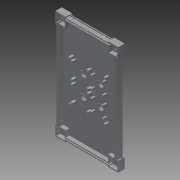
# Autodesk Inventor part: SimpleLensPlane
Saved by Autodesk Inventor 2015 (Build 190159000, 159)
## iProperties
Created: 2015-03-20
Part Number: SimpleLensPlane
Material: NylonD2W
Document SubType Name: Modeling
Designer: Akovo_000
Density: 0.93 g/cm^3
Appearance: Nylon 6
Mass: 59.4864 g
Surface Area: 763.227 cm^2
Volume: 63.9639 cm^3
Author: Akovo_000
Autodesk Inventor part; units mm, degrees
ref_plane "YZ Plane" through (0, 0, 0) normal (1, 0, 0) x (0, 1, 0)
ref_plane "XZ Plane" through (0, 0, 0) normal (0, 1, 0) x (-1, 0, 0)
ref_plane "XY Plane" through (0, 0, 0) normal (0, 0, 1) x (1, 0, 0)
ref_plane "Main Work Pane" through (0, 2.75, 7) normal (0, 1, 0) x (-1, 0, 0)
sketch "Panel" plane through (0, 2.75, 7) normal (0, 1, 0) x (-1, 0, 0)
  circle A0 centre (9.4297, 27.3549) radius 5.8
  circle A1 centre (9.4297, -11.6451) radius 5.8
  circle A2 centre (43.2297, -11.6451) radius 5.8
  circle A3 centre (43.2297, 27.3549) radius 5.8
  line L0 (43.2297, -11.6451) -> (43.2297, -11.6451)
  line L1 (61.2297, 45.3549) -> (25.2297, 45.3549)
  line L2 (25.2297, 45.3549) -> (25.2297, 9.3549)
  line L3 (25.2297, 9.3549) -> (61.2297, 9.3549)
  line L4 (61.2297, 9.3549) -> (61.2297, 45.3549)
  line L5 (61.2297, 45.3549) -> (25.2297, 9.3549) construction
  line L6 (25.2297, 45.3549) -> (61.2297, 9.3549) construction
  line L7 (61.2297, 6.3549) -> (25.2297, 6.3549)
  line L8 (25.2297, 6.3549) -> (25.2297, -29.6451)
  line L9 (25.2297, -29.6451) -> (61.2297, -29.6451)
  line L10 (61.2297, -29.6451) -> (61.2297, 6.3549)
  line L11 (61.2297, 6.3549) -> (25.2297, -29.6451) construction
  line L12 (25.2297, 6.3549) -> (61.2297, -29.6451) construction
  line L13 (22.2297, 40.1549) -> (-3.3703, 40.1549)
  line L14 (-3.3703, 40.1549) -> (-3.3703, 14.5549)
  line L15 (-3.3703, 14.5549) -> (22.2297, 14.5549)
  line L16 (22.2297, 14.5549) -> (22.2297, 40.1549)
  line L17 (22.2297, 40.1549) -> (-3.3703, 14.5549) construction
  line L18 (-3.3703, 40.1549) -> (22.2297, 14.5549) construction
  line L19 (22.2297, 1.1549) -> (-3.3703, 1.1549)
  line L20 (-3.3703, 1.1549) -> (-3.3703, -24.4451)
  line L21 (-3.3703, -24.4451) -> (22.2297, -24.4451)
  line L22 (22.2297, -24.4451) -> (22.2297, 1.1549)
  line L23 (22.2297, 1.1549) -> (-3.3703, -24.4451) construction
  line L24 (-3.3703, 1.1549) -> (22.2297, -24.4451) construction
  line L25 (61.2297, -29.6451) -> (61.2297, 45.3549)
  line L26 (61.2297, 45.3549) -> (-3.3703, 45.3549)
  line L27 (-3.3703, 45.3549) -> (-3.3703, -29.6451)
  line L28 (-3.3703, -29.6451) -> (61.2297, -29.6451)
  line L29 (90.0297, -97.7451) -> (-32.1703, -97.7451)
  line L30 (-32.1703, -97.7451) -> (-32.1703, 113.4549)
  line L31 (-32.1703, 113.4549) -> (90.0297, 113.4549)
  line L32 (90.0297, 113.4549) -> (90.0297, -97.7451)
  line L33 (43.2297, 21.5549) -> (43.2297, -5.8451) construction
  line L34 (37.4297, 27.3549) -> (15.2297, 27.3549) construction
  line L35 (9.4297, 21.5549) -> (9.4297, -5.8451) construction
  line L36 (15.2297, -11.6451) -> (37.4297, -11.6451) construction
  line L37 (17.4252, 113.4549) -> (17.4252, 45.3549) construction
  line L38 (17.4252, -29.6451) -> (17.4252, -97.7451) construction
  line L39 (61.2297, 7.8549) -> (90.0297, 7.8549) construction
  line L40 (-3.3703, 7.8549) -> (-32.1703, 7.8549) construction
  line L41 (71.9297, 95.3549) -> (88.0297, 95.3549)
  line L42 (88.0297, 95.3549) -> (88.0297, 111.4549)
  line L43 (88.0297, 111.4549) -> (71.9297, 111.4549)
  line L44 (71.9297, 111.4549) -> (71.9297, 95.3549)
  line L45 (69.9297, 113.4549) -> (69.9297, 93.3549)
  line L46 (69.9297, 93.3549) -> (90.0297, 93.3549)
  line L47 (88.0297, -95.7451) -> (71.9297, -95.7451)
  line L48 (71.9297, -95.7451) -> (71.9297, -79.6451)
  line L49 (71.9297, -79.6451) -> (88.0297, -79.6451)
  line L50 (88.0297, -79.6451) -> (88.0297, -95.7451)
  line L51 (90.0297, -77.6451) -> (69.9297, -77.6451)
  line L52 (69.9297, -77.6451) -> (69.9297, -97.7451)
  line L53 (-30.1703, -95.7451) -> (-14.0703, -95.7451)
  line L54 (-14.0703, -95.7451) -> (-14.0703, -79.6451)
  line L55 (-14.0703, -79.6451) -> (-30.1703, -79.6451)
  line L56 (-30.1703, -79.6451) -> (-30.1703, -95.7451)
  line L57 (-12.0703, -97.7451) -> (-12.0703, -77.6451)
  line L58 (-12.0703, -77.6451) -> (-32.1703, -77.6451)
  line L59 (-14.0703, 95.3549) -> (-30.1703, 95.3549)
  line L60 (-30.1703, 95.3549) -> (-30.1703, 111.4549)
  line L61 (-30.1703, 111.4549) -> (-14.0703, 111.4549)
  line L62 (-14.0703, 111.4549) -> (-14.0703, 95.3549)
  line L63 (-12.0703, 113.4549) -> (-12.0703, 93.3549)
  line L64 (-12.0703, 93.3549) -> (-32.1703, 93.3549)
  circle A4 centre (76.9297, 100.3549) radius 2
  circle A5 centre (-19.0703, 100.3549) radius 2
  circle A6 centre (76.9297, -84.6451) radius 2
  circle A7 centre (-19.0703, -84.6451) radius 2
  line L65 (69.9297, 93.3549) -> (69.9297, -77.6451)
  line L66 (69.9297, -77.6451) -> (-12.0703, -77.6451)
  line L67 (-12.0703, -77.6451) -> (-12.0703, 93.3549)
  line L68 (-12.0703, 93.3549) -> (69.9297, 93.3549)
  line L69 (-19.0703, -84.6451) -> (-14.0703, -84.6451) construction
  line L70 (-19.0703, -84.6451) -> (-19.0703, -79.6451) construction
  line L71 (76.9297, -84.6451) -> (71.9297, -84.6451) construction
  line L72 (76.9297, -84.6451) -> (76.9297, -79.6451) construction
  line L73 (76.9297, 100.3549) -> (76.9297, 95.3549) construction
  line L74 (76.9297, 100.3549) -> (71.9297, 100.3549) construction
  line L75 (-19.0703, 100.3549) -> (-14.0703, 100.3549) construction
  line L76 (-19.0703, 100.3549) -> (-19.0703, 95.3549) construction
  dimension "d337" = 11.6
  dimension "d490" = 36
  dimension "d491" = 36
  dimension "d494" = 3
  dimension "d495" = 25.6
  dimension "d496" = 25.6
  dimension "d497" = 3
  dimension "d498" = 0
  dimension "d584" = 2
  dimension "d585" = 2
  dimension "d586" = 2
  dimension "d587" = 2
  dimension "d588" = 16.1
  dimension "d589" = 16.1
  dimension "d592" = 2
  dimension "d593" = 4
  dimension "d597" = 2
  dimension "d648" = 2
  dimension "d661" = 5
  dimension "d670" = 175
  dimension "d671" = 86
  constraints: 154 end point, 30 perpendicular, 21 equal length, 20 parallel, 20 point on line, 12 collinear, 12 midpoint, 11 horizontal, 8 centre point, 8 point on circle, 6 equal radius, 6 line through centre, 5 vertical
  measures "d337" diameter of A2
  measures "d490" distance of L3.end L2.end
  measures "d491" distance of L2.end L1.end
  measures "d494" distance between parallel lines of L7 L3
  measures "d495" distance of L15.end L14.end
  measures "d496" distance of L14.end L13.end
  measures "d497" distance between parallel lines of L22 L8
  measures "d498" distance between parallel lines of L27 L14
  measures "d584" distance between parallel lines of L31 L43
  measures "d585" distance between parallel lines of L32 L42
  measures "d586" distance between parallel lines of L46 L41
  measures "d587" distance between parallel lines of L44 L45
  measures "d588" distance between parallel lines of L41 L43
  measures "d589" distance between parallel lines of L42 L44
  measures "d592" distance between parallel lines of L30 L56
  measures "d593" diameter of A4
  measures "d597" distance between parallel lines of L29 L47
  measures "d648" distance between parallel lines of L62 L63
  measures "d661" distance of L69.start L70.end
  measures "d670" distance between parallel lines of L49 L41
  measures "d671" distance between parallel lines of L44 L62
extrude "FlatPlane" add sketch "Panel" along normal blind 1.5 contours L4 L3 L2 L1 | L2 L3 L25 L7 L8 L28 L27 L21 L22 L19 L15 L16 L13 L26 | L10 L9 L8 L7 | L13 L16 L15 L14 | L19 L22 L21 L20 | L29 L52 L51 L32 | L29 L57 L66 L52 | L51 L65 L46 L32 | L29 L30 L58 L57 | L66 L67 L68 L65 | L46 L45 L31 L32 | L58 L30 L64 L67 | L68 L63 L31 L45 | L64 L30 L31 L63 | L44 L43 L42 L41 | L47 L48 L49 L50 | L56 L55 L54 L53 | L59 L60 L61 L62
sketch "BoardSuport" plane through (0, 2.75, 7) normal (0, -1, 0) x (1, 0, 0)
  line L0 (-58.7297, 42.8549) -> (-27.7297, 42.8549) construction
  line L1 (-27.7297, 42.8549) -> (-27.7297, 11.8549) construction
  line L2 (-27.7297, 11.8549) -> (-58.7297, 11.8549) construction
  line L3 (-58.7297, 11.8549) -> (-58.7297, 42.8549) construction
  circle A0 centre (-43.2297, 27.3549) radius 5.8
  line L4 (-58.7297, 42.8549) -> (-27.7297, 11.8549) construction
  line L5 (-27.7297, 42.8549) -> (-58.7297, 11.8549) construction
  line L6 (-58.7297, 3.8549) -> (-27.7297, 3.8549) construction
  line L7 (-27.7297, 3.8549) -> (-27.7297, -27.1451) construction
  line L8 (-27.7297, -27.1451) -> (-58.7297, -27.1451) construction
  line L9 (-58.7297, -27.1451) -> (-58.7297, 3.8549) construction
  circle A1 centre (-43.2297, -11.6451) radius 5.8
  line L10 (-58.7297, 3.8549) -> (-27.7297, -27.1451) construction
  line L11 (-27.7297, 3.8549) -> (-58.7297, -27.1451) construction
  line L12 (-20.6797, 38.6049) -> (1.8203, 38.6049) construction
  line L13 (1.8203, 38.6049) -> (1.8203, 16.1049) construction
  line L14 (1.8203, 16.1049) -> (-20.6797, 16.1049) construction
  line L15 (-20.6797, 16.1049) -> (-20.6797, 38.6049) construction
  circle A2 centre (-9.4297, 27.3549) radius 5.8
  line L16 (-20.6797, 38.6049) -> (1.8203, 16.1049) construction
  line L17 (1.8203, 38.6049) -> (-20.6797, 16.1049) construction
  line L18 (-20.6797, -0.3951) -> (1.8203, -0.3951) construction
  line L19 (1.8203, -0.3951) -> (1.8203, -22.8951) construction
  line L20 (1.8203, -22.8951) -> (-20.6797, -22.8951) construction
  line L21 (-20.6797, -22.8951) -> (-20.6797, -0.3951) construction
  circle A3 centre (-9.4297, -11.6451) radius 5.8
  line L22 (-20.6797, -0.3951) -> (1.8203, -22.8951) construction
  line L23 (1.8203, -0.3951) -> (-20.6797, -22.8951) construction
  line L24 (-60.8297, 5.9549) -> (-56.6297, 5.9549)
  line L25 (-56.6297, 5.9549) -> (-56.6297, 1.7549)
  line L26 (-56.6297, 1.7549) -> (-60.8297, 1.7549)
  line L27 (-60.8297, 1.7549) -> (-60.8297, 5.9549)
  line L28 (-60.8297, 5.9549) -> (-56.6297, 1.7549) construction
  line L29 (-56.6297, 5.9549) -> (-60.8297, 1.7549) construction
  line L30 (-60.8297, 13.9549) -> (-56.6297, 13.9549)
  line L31 (-56.6297, 13.9549) -> (-56.6297, 9.7549)
  line L32 (-56.6297, 9.7549) -> (-60.8297, 9.7549)
  line L33 (-60.8297, 9.7549) -> (-60.8297, 13.9549)
  line L34 (-60.8297, 13.9549) -> (-56.6297, 9.7549) construction
  line L35 (-56.6297, 13.9549) -> (-60.8297, 9.7549) construction
  line L36 (-29.8297, 13.9549) -> (-25.6297, 13.9549)
  line L37 (-25.6297, 13.9549) -> (-25.6297, 9.7549)
  line L38 (-25.6297, 9.7549) -> (-29.8297, 9.7549)
  line L39 (-29.8297, 9.7549) -> (-29.8297, 13.9549)
  line L40 (-29.8297, 13.9549) -> (-25.6297, 9.7549) construction
  line L41 (-25.6297, 13.9549) -> (-29.8297, 9.7549) construction
  line L42 (-29.8297, 44.9549) -> (-25.6297, 44.9549)
  line L43 (-25.6297, 44.9549) -> (-25.6297, 40.7549)
  line L44 (-25.6297, 40.7549) -> (-29.8297, 40.7549)
  line L45 (-29.8297, 40.7549) -> (-29.8297, 44.9549)
  line L46 (-29.8297, 44.9549) -> (-25.6297, 40.7549) construction
  line L47 (-25.6297, 44.9549) -> (-29.8297, 40.7549) construction
  line L48 (-60.8297, 44.9549) -> (-56.6297, 44.9549)
  line L49 (-56.6297, 44.9549) -> (-56.6297, 40.7549)
  line L50 (-56.6297, 40.7549) -> (-60.8297, 40.7549)
  line L51 (-60.8297, 40.7549) -> (-60.8297, 44.9549)
  line L52 (-60.8297, 44.9549) -> (-56.6297, 40.7549) construction
  line L53 (-56.6297, 44.9549) -> (-60.8297, 40.7549) construction
  line L54 (-29.8297, 5.9549) -> (-25.6297, 5.9549)
  line L55 (-25.6297, 5.9549) -> (-25.6297, 1.7549)
  line L56 (-25.6297, 1.7549) -> (-29.8297, 1.7549)
  line L57 (-29.8297, 1.7549) -> (-29.8297, 5.9549)
  line L58 (-29.8297, 5.9549) -> (-25.6297, 1.7549) construction
  line L59 (-25.6297, 5.9549) -> (-29.8297, 1.7549) construction
  line L60 (-29.8297, -25.0451) -> (-25.6297, -25.0451)
  line L61 (-25.6297, -25.0451) -> (-25.6297, -29.2451)
  line L62 (-25.6297, -29.2451) -> (-29.8297, -29.2451)
  line L63 (-29.8297, -29.2451) -> (-29.8297, -25.0451)
  line L64 (-29.8297, -25.0451) -> (-25.6297, -29.2451) construction
  line L65 (-25.6297, -25.0451) -> (-29.8297, -29.2451) construction
  line L66 (-60.8297, -25.0451) -> (-56.6297, -25.0451)
  line L67 (-56.6297, -25.0451) -> (-56.6297, -29.2451)
  line L68 (-56.6297, -29.2451) -> (-60.8297, -29.2451)
  line L69 (-60.8297, -29.2451) -> (-60.8297, -25.0451)
  line L70 (-60.8297, -25.0451) -> (-56.6297, -29.2451) construction
  line L71 (-56.6297, -25.0451) -> (-60.8297, -29.2451) construction
  line L72 (-22.1797, -21.3951) -> (-19.1797, -21.3951)
  line L73 (-19.1797, -21.3951) -> (-19.1797, -24.3951)
  line L74 (-19.1797, -24.3951) -> (-22.1797, -24.3951)
  line L75 (-22.1797, -24.3951) -> (-22.1797, -21.3951)
  line L76 (-22.1797, -21.3951) -> (-19.1797, -24.3951) construction
  line L77 (-19.1797, -21.3951) -> (-22.1797, -24.3951) construction
  line L78 (0.3203, -21.3951) -> (3.3203, -21.3951)
  line L79 (3.3203, -21.3951) -> (3.3203, -24.3951)
  line L80 (3.3203, -24.3951) -> (0.3203, -24.3951)
  line L81 (0.3203, -24.3951) -> (0.3203, -21.3951)
  line L82 (0.3203, -21.3951) -> (3.3203, -24.3951) construction
  line L83 (3.3203, -21.3951) -> (0.3203, -24.3951) construction
  line L84 (0.3203, 1.1049) -> (3.3203, 1.1049)
  line L85 (3.3203, 1.1049) -> (3.3203, -1.8951)
  line L86 (3.3203, -1.8951) -> (0.3203, -1.8951)
  line L87 (0.3203, -1.8951) -> (0.3203, 1.1049)
  line L88 (0.3203, 1.1049) -> (3.3203, -1.8951) construction
  line L89 (3.3203, 1.1049) -> (0.3203, -1.8951) construction
  line L90 (-22.1797, 1.1049) -> (-19.1797, 1.1049)
  line L91 (-19.1797, 1.1049) -> (-19.1797, -1.8951)
  line L92 (-19.1797, -1.8951) -> (-22.1797, -1.8951)
  line L93 (-22.1797, -1.8951) -> (-22.1797, 1.1049)
  line L94 (-22.1797, 1.1049) -> (-19.1797, -1.8951) construction
  line L95 (-19.1797, 1.1049) -> (-22.1797, -1.8951) construction
  line L96 (-22.1797, 14.6049) -> (-19.1797, 14.6049)
  line L97 (-19.1797, 14.6049) -> (-19.1797, 17.6049)
  line L98 (-19.1797, 17.6049) -> (-22.1797, 17.6049)
  line L99 (-22.1797, 17.6049) -> (-22.1797, 14.6049)
  line L100 (-22.1797, 14.6049) -> (-19.1797, 17.6049) construction
  line L101 (-19.1797, 14.6049) -> (-22.1797, 17.6049) construction
  line L102 (3.3203, 14.6049) -> (0.3203, 14.6049)
  line L103 (0.3203, 14.6049) -> (0.3203, 17.6049)
  line L104 (0.3203, 17.6049) -> (3.3203, 17.6049)
  line L105 (3.3203, 17.6049) -> (3.3203, 14.6049)
  line L106 (3.3203, 14.6049) -> (0.3203, 17.6049) construction
  line L107 (0.3203, 14.6049) -> (3.3203, 17.6049) construction
  line L108 (3.3203, 40.1049) -> (0.3203, 40.1049)
  line L109 (0.3203, 40.1049) -> (0.3203, 37.1049)
  line L110 (0.3203, 37.1049) -> (3.3203, 37.1049)
  line L111 (3.3203, 37.1049) -> (3.3203, 40.1049)
  line L112 (3.3203, 40.1049) -> (0.3203, 37.1049) construction
  line L113 (0.3203, 40.1049) -> (3.3203, 37.1049) construction
  line L114 (-22.1797, 40.1049) -> (-19.1797, 40.1049)
  line L115 (-19.1797, 40.1049) -> (-19.1797, 37.1049)
  line L116 (-19.1797, 37.1049) -> (-22.1797, 37.1049)
  line L117 (-22.1797, 37.1049) -> (-22.1797, 40.1049)
  line L118 (-22.1797, 40.1049) -> (-19.1797, 37.1049) construction
  line L119 (-19.1797, 40.1049) -> (-22.1797, 37.1049) construction
  arc A4 (-58.7297, 40.7549) -> (-56.6297, 42.8549) centre (-58.7297, 42.8549) ccw
  arc A5 (-29.8297, 42.8549) -> (-27.7297, 40.7549) centre (-27.7297, 42.8549) ccw
  arc A6 (-27.7297, 13.9549) -> (-29.8297, 11.8549) centre (-27.7297, 11.8549) ccw
  arc A7 (-56.6297, 11.8549) -> (-58.7297, 13.9549) centre (-58.7297, 11.8549) ccw
  arc A8 (-58.7297, 1.7549) -> (-56.6297, 3.8549) centre (-58.7297, 3.8549) ccw
  arc A9 (-56.6297, -27.1451) -> (-58.7297, -25.0451) centre (-58.7297, -27.1451) ccw
  arc A10 (-27.7297, -25.0451) -> (-29.8297, -27.1451) centre (-27.7297, -27.1451) ccw
  arc A11 (-19.1797, -22.8951) -> (-20.6797, -21.3951) centre (-20.6797, -22.8951) ccw
  arc A12 (1.8203, -21.3951) -> (0.3203, -22.8951) centre (1.8203, -22.8951) ccw
  arc A13 (0.3203, -0.3951) -> (1.8203, -1.8951) centre (1.8203, -0.3951) ccw
  arc A14 (-20.6797, -1.8951) -> (-19.1797, -0.3951) centre (-20.6797, -0.3951) ccw
  arc A15 (-29.8297, 3.8549) -> (-27.7297, 1.7549) centre (-27.7297, 3.8549) ccw
  arc A16 (-20.6797, 37.1049) -> (-19.1797, 38.6049) centre (-20.6797, 38.6049) ccw
  arc A17 (-19.1797, 16.1049) -> (-20.6797, 17.6049) centre (-20.6797, 16.1049) ccw
  arc A18 (1.8203, 17.6049) -> (0.3203, 16.1049) centre (1.8203, 16.1049) ccw
  arc A19 (0.3203, 38.6049) -> (1.8203, 37.1049) centre (1.8203, 38.6049) ccw
  circle A20 centre (-58.7297, 42.8549) radius 0.9
  circle A21 centre (-58.7297, 11.8549) radius 0.9
  circle A22 centre (-27.7297, 11.8549) radius 0.9
  circle A23 centre (-27.7297, 42.8549) radius 0.9
  circle A24 centre (-58.7297, 3.8549) radius 0.9
  circle A25 centre (-58.7297, -27.1451) radius 0.9
  circle A26 centre (-27.7297, -27.1451) radius 0.9
  circle A27 centre (-27.7297, 3.8549) radius 0.9
  circle A28 centre (-20.6797, -0.3951) radius 0.9
  circle A29 centre (-20.6797, -22.8951) radius 0.9
  circle A30 centre (1.8203, -22.8951) radius 0.9
  circle A31 centre (1.8203, -0.3951) radius 0.9
  circle A32 centre (1.8203, 16.1049) radius 0.9
  circle A33 centre (-20.6797, 16.1049) radius 0.9
  circle A34 centre (1.8203, 38.6049) radius 0.9
  circle A35 centre (-20.6797, 38.6049) radius 0.9
  line L120 (-90.0297, 113.4549) -> (-69.8297, 113.4549)
  line L121 (-69.8297, 113.4549) -> (-69.8297, 111.4549)
  line L122 (-69.8297, 93.2549) -> (-82.0297, 93.2549)
  line L123 (-90.0297, 93.2549) -> (-90.0297, 113.4549)
  line L124 (32.1703, 113.4549) -> (11.9703, 113.4549)
  line L125 (11.9703, 113.4549) -> (11.9703, 111.4549)
  line L126 (11.9703, 93.2549) -> (24.1703, 93.2549)
  line L127 (32.1703, 93.2549) -> (32.1703, 113.4549)
  line L128 (-90.0297, -97.7451) -> (-69.8297, -97.7451)
  line L129 (-69.8297, -97.7451) -> (-69.8297, -77.5451)
  line L130 (-69.8297, -77.5451) -> (-82.0297, -77.5451)
  line L131 (-90.0297, -77.5451) -> (-90.0297, -97.7451)
  line L132 (32.1703, -97.7451) -> (11.9703, -97.7451)
  line L133 (11.9703, -97.7451) -> (11.9703, -95.7451)
  line L134 (11.9703, -77.5451) -> (24.1703, -77.5451)
  line L135 (32.1703, -77.5451) -> (32.1703, -97.7451)
  line L136 (-90.0297, 93.2549) -> (-88.0297, 93.2549)
  line L137 (-82.0297, 93.2549) -> (-82.0297, -77.5451)
  line L138 (-82.0297, -77.5451) -> (-88.0297, -77.5451)
  line L139 (-90.0297, -77.5451) -> (-90.0297, 93.2549) construction
  line L140 (-69.8297, -97.7451) -> (11.9703, -97.7451) construction
  line L141 (11.9703, -97.7451) -> (11.9703, -89.7451)
  line L142 (11.9703, -89.7451) -> (-69.8297, -89.7451)
  line L143 (-69.8297, -89.7451) -> (-69.8297, -97.7451)
  line L144 (32.1703, -77.5451) -> (30.1703, -77.5451)
  line L145 (24.1703, -77.5451) -> (24.1703, 93.2549)
  line L146 (24.1703, 93.2549) -> (30.1703, 93.2549)
  line L147 (32.1703, 93.2549) -> (32.1703, -77.5451) construction
  line L148 (11.9703, 113.4549) -> (-69.8297, 113.4549) construction
  line L149 (-69.8297, 113.4549) -> (-69.8297, 111.4549)
  line L150 (-69.8297, 105.4549) -> (11.9703, 105.4549)
  line L151 (11.9703, 105.4549) -> (11.9703, 111.4549)
  circle A36 centre (-43.2297, 27.3549) radius 5.8 projected
  circle A37 centre (-9.4297, 27.3549) radius 5.8 projected
  circle A38 centre (-43.2297, -11.6451) radius 5.8 projected
  circle A39 centre (-9.4297, -11.6451) radius 5.8 projected
  line L152 (11.9703, -95.7451) -> (-69.8297, -95.7451)
  line L153 (-88.0297, -77.5451) -> (-88.0297, -73.7451)
  line L154 (11.9703, 111.4549) -> (-69.8297, 111.4549)
  line L155 (32.1703, -97.7451) -> (-90.0297, -97.7451) projected
  line L156 (30.1703, -77.5451) -> (30.1703, 93.2549)
  line L157 (-82.0297, -77.5451) -> (-88.0297, -77.5451)
  line L158 (-88.0297, -77.5451) -> (-90.0297, -77.5451)
  line L159 (-69.8297, 105.4549) -> (-69.8297, 93.2549)
  line L160 (-69.8297, 111.4549) -> (-69.8297, 105.4549)
  line L161 (24.1703, 93.2549) -> (30.1703, 93.2549)
  line L162 (30.1703, 93.2549) -> (32.1703, 93.2549)
  line L163 (11.9703, -95.7451) -> (11.9703, -89.7451)
  line L164 (11.9703, -89.7451) -> (11.9703, -77.5451)
  line L165 (30.1703, 93.2549) -> (32.1703, 93.2549)
  line L166 (-88.0297, -73.7451) -> (-88.0297, 93.2549)
  line L167 (-88.0297, 93.2549) -> (-90.0297, 93.2549)
  line L168 (-82.0297, 93.2549) -> (-88.0297, 93.2549)
  line L169 (11.9703, 105.4549) -> (11.9703, 93.2549)
  line L170 (11.9703, 111.4549) -> (11.9703, 105.4549)
  line L171 (30.1703, -77.5451) -> (24.1703, -77.5451)
  line L172 (24.1703, -77.5451) -> (32.1703, -77.5451)
  line L173 (-88.0297, -77.5451) -> (-90.0297, -77.5451)
  line L174 (-88.0297, 93.2549) -> (-82.0297, 93.2549)
  line L175 (11.9703, 111.4549) -> (11.9703, 113.4549)
  line L176 (-69.8297, 111.4549) -> (-69.8297, 105.4549)
  line L177 (-60.8297, 44.9549) -> (3.3203, 44.9549) construction
  line L178 (3.3203, 44.9549) -> (3.3203, -29.2451) construction
  line L179 (3.3203, -29.2451) -> (-60.8297, -29.2451) construction
  line L180 (-60.8297, -29.2451) -> (-60.8297, 44.9549) construction
  line L181 (-60.8297, 44.9549) -> (-64.8297, 44.9549)
  line L182 (-64.8297, 44.9549) -> (-64.8297, 48.9549)
  line L183 (-64.8297, 48.9549) -> (-60.8297, 48.9549)
  line L184 (-60.8297, 48.9549) -> (-60.8297, 44.9549)
  line L185 (-60.8297, -29.2451) -> (-64.8297, -29.2451)
  line L186 (-64.8297, -29.2451) -> (-64.8297, -33.2451)
  line L187 (-64.8297, -33.2451) -> (-60.8297, -33.2451)
  line L188 (-60.8297, -33.2451) -> (-60.8297, -29.2451)
  line L189 (3.3203, -29.2451) -> (7.3203, -29.2451)
  line L190 (7.3203, -29.2451) -> (7.3203, -33.2451)
  line L191 (7.3203, -33.2451) -> (3.3203, -33.2451)
  line L192 (3.3203, -33.2451) -> (3.3203, -29.2451)
  line L193 (3.3203, 44.9549) -> (7.3203, 44.9549)
  line L194 (7.3203, 44.9549) -> (7.3203, 48.9549)
  line L195 (7.3203, 48.9549) -> (3.3203, 48.9549)
  line L196 (3.3203, 48.9549) -> (3.3203, 44.9549)
  circle A40 centre (5.4519, 46.9805) radius 0.9
  circle A41 centre (-62.6981, 46.9805) radius 0.9
  circle A42 centre (-62.6981, -31.2195) radius 0.9
  circle A43 centre (5.4519, -31.2195) radius 0.9
  dimension "d543" = 22.5
  dimension "d545" = 4.2
  dimension "d546" = 3
  dimension "d547" = 1.8
  dimension "d548" = 1.8
  dimension "d617" = 20.2
  dimension "d642" = 31
  dimension "d643" = 31
  dimension "d644" = 22.5
  dimension "d645" = 0
  dimension "d646" = 0
  dimension "d647" = 11.6
  dimension "d658" = 2
  dimension "d659" = 6
  dimension "d660" = 20.2
  dimension "d662" = 4
  dimension "d665" = 72.15
  dimension "d666" = 82.2
  dimension "d667" = 1.8
  constraints: 392 end point, 93 parallel, 76 midpoint, 42 perpendicular, 40 centre point, 35 horizontal, 34 equal length, 32 point on circle, 24 point on line, 20 equal radius, 16 tangent, 15 coincident, 3 concentric
  measures "d543" distance of L12.end L13.end
  measures "d545" distance between parallel lines of L24 L26
  measures "d546" distance between parallel lines of L80 L78
  measures "d547" diameter of A25
  measures "d548" diameter of A30
  measures "d617" distance of L132.end L134.start
  measures "d642" distance of L0.end L0.start
  measures "d643" distance of L2.end L0.start
  measures "d644" distance of L12.start L12.end
  measures "d645" distance of A0.centre A36.centre
  measures "d646" distance of A36.centre A0.centre
  measures "d647" diameter of A0
  measures "d658" distance between parallel lines of L155 L152
  measures "d659" distance between parallel lines of L152 L142
  measures "d660" distance of L132.end L132.start
  measures "d662" distance of L182.end L183.end
  measures "d665" distance between parallel lines of L186 L190
  measures "d666" distance between parallel lines of L195 L191
  measures "d667" diameter of A40
extrude "BoardSupport3D" add sketch "BoardSuport" along normal blind 7.2 contours L24 L25 A8 L26 L27 | L25 L26 A8 | L30 A7 L31 L32 L33 | L30 L31 A7 | L36 A6 L39 | L36 L37 L38 L39 A6 | L42 L43 L44 A5 L45 | A5 L44 L45 | L48 L49 A4 L50 L51 | L181 L182 L183 L184 | L49 L50 A4 | L54 L55 L56 A15 L57 | A15 L56 L57 | L60 A10 L63 | L60 L61 L62 L63 A10 | L188 L187 L186 L185 | L66 A9 L67 L68 L69 | L66 L67 A9 | L72 A11 L73 L74 L75 | L72 L73 A11 | L78 A12 L81 | L78 L79 L80 L81 A12 | L84 L85 L86 A13 L87 | A13 L86 L87 | L90 L91 A14 L92 L93 | L91 L92 A14 | L99 L98 A17 L97 L96 | A17 L98 L97 | L102 L103 A18 L104 L105 | L103 L104 A18 | L111 L110 A19 L109 L108 | A19 L110 L109 | L114 L115 A16 L116 L117 | L115 L116 A16 | L120 L121 L160 L159 L122 L168 L136 L123 | L154 L151 L150 L160 | L168 L137 L138 L153 L166 | L125 L124 L127 L162 L146 L126 L169 L151 | L138 L130 L129 L128 L131 L158 | L146 L156 L171 L145 | L142 L141 L152 L129 | L171 L144 L135 L132 L133 L141 L164 L134 | L189 L190 L191 L192 | L196 L195 L194 L193
sketch "Lens and screwcover" plane through (0, 4.25, 7) normal (0, 1, 0) x (1, 0, 0)
  circle A0 centre (-43.2297, -27.3549) radius 5.8
  circle A1 centre (-43.2297, -27.3549) radius 5.8
  circle A2 centre (-9.4297, -27.3549) radius 5.8
  circle A3 centre (-9.4297, -27.3549) radius 5.8
  circle A4 centre (-9.4297, 11.6451) radius 5.8
  circle A5 centre (-9.4297, 11.6451) radius 5.8
  circle A6 centre (-43.2297, 11.6451) radius 5.8
  circle A7 centre (-43.2297, 11.6451) radius 5.8
  circle A8 centre (-43.2297, -27.3549) radius 8.3
  circle A9 centre (-9.4297, -27.3549) radius 8.3
  circle A10 centre (-9.4297, 11.6451) radius 8.3
  circle A11 centre (-43.2297, 11.6451) radius 8.3
  line L0 (32.1703, 97.7451) -> (11.9703, 97.7451)
  line L1 (11.9703, 97.7451) -> (11.9703, 77.5451)
  line L2 (11.9703, 77.5451) -> (32.1703, 77.5451)
  line L3 (32.1703, 77.5451) -> (32.1703, 97.7451)
  line L4 (-90.0297, 97.7451) -> (-69.8297, 97.7451)
  line L5 (-69.8297, 97.7451) -> (-69.8297, 77.5451)
  line L6 (-69.8297, 77.5451) -> (-90.0297, 77.5451)
  line L7 (-90.0297, 77.5451) -> (-90.0297, 97.7451)
  line L8 (-90.0297, -113.4549) -> (-69.8297, -113.4549)
  line L9 (-69.8297, -113.4549) -> (-69.8297, -93.2549)
  line L10 (-69.8297, -93.2549) -> (-90.0297, -93.2549)
  line L11 (-90.0297, -93.2549) -> (-90.0297, -113.4549)
  line L12 (32.1703, -113.4549) -> (11.9703, -113.4549)
  line L13 (11.9703, -113.4549) -> (11.9703, -93.2549)
  line L14 (11.9703, -93.2549) -> (32.1703, -93.2549)
  line L15 (32.1703, -93.2549) -> (32.1703, -113.4549)
  circle A12 centre (-43.2297, -27.3549) radius 5.8 projected
  circle A13 centre (-43.2297, 11.6451) radius 5.8 projected
  circle A14 centre (-9.4297, 11.6451) radius 5.8 projected
  circle A15 centre (-9.4297, -27.3549) radius 5.8 projected
  circle A16 centre (-76.9297, 84.6451) radius 2 projected
  circle A17 centre (-76.9297, 84.6451) radius 2
  circle A18 centre (19.0703, 84.6451) radius 2 projected
  circle A19 centre (19.0703, 84.6451) radius 2
  circle A20 centre (19.0703, -100.3549) radius 2 projected
  circle A21 centre (19.0703, -100.3549) radius 2
  circle A22 centre (-76.9297, -100.3549) radius 2 projected
  circle A23 centre (-76.9297, -100.3549) radius 2
  point P0 (0, 7)
  dimension "d551" = 2.5
  dimension "d600" = 20.2
  dimension "d601" = 20.2
  constraints: 32 end point, 16 centre point, 12 coincident, 8 parallel, 6 equal length, 4 concentric, 4 horizontal, 4 perpendicular, 3 equal radius, 2 point on line
  measures "d551" radial gap between concentric circles of A8 A0
  measures "d600" distance of L2.end L1.end
  measures "d601" distance of L1.end L0.end
extrude "Extrusion15" add sketch "Lens and screwcover" along normal blind 3.5
sketch "Sketch20" plane through (0, -4.45, 7) normal (0, -1, 0) x (1, 0, 0)
  line L0 (32.1703, 93.2549) -> (32.1703, 113.4549)
  line L1 (32.1703, 113.4549) -> (11.9703, 113.4549)
  line L2 (-69.8297, 93.2549) -> (-90.0297, 93.2549)
  line L3 (-90.0297, 93.2549) -> (-90.0297, 113.4549)
  line L4 (-90.0297, 113.4549) -> (-69.8297, 113.4549)
  line L5 (-69.8297, 113.4549) -> (-69.8297, 93.2549)
  line L6 (32.1703, -97.7451) -> (11.9703, -97.7451)
  line L7 (11.9703, -97.7451) -> (11.9703, -77.5451)
  line L8 (11.9703, -77.5451) -> (32.1703, -77.5451)
  line L9 (32.1703, -77.5451) -> (32.1703, -97.7451)
  line L10 (-69.8297, -77.5451) -> (-90.0297, -77.5451)
  line L11 (-90.0297, -77.5451) -> (-90.0297, -97.7451)
  line L12 (-90.0297, -97.7451) -> (-69.8297, -97.7451)
  line L13 (-69.8297, -97.7451) -> (-69.8297, -77.5451)
  line L14 (13.9703, 95.2549) -> (30.1703, 95.2549)
  line L15 (30.1703, 95.2549) -> (30.1703, 111.4549)
  line L16 (30.1703, 111.4549) -> (13.9703, 111.4549)
  line L17 (13.9703, 111.4549) -> (13.9703, 95.2549)
  line L18 (-71.8297, 95.2549) -> (-88.0297, 95.2549)
  line L19 (-88.0297, 95.2549) -> (-88.0297, 111.4549)
  line L20 (-88.0297, 111.4549) -> (-71.8297, 111.4549)
  line L21 (-71.8297, 111.4549) -> (-71.8297, 95.2549)
  line L22 (-88.0297, -95.7451) -> (-71.8297, -95.7451)
  line L23 (-71.8297, -95.7451) -> (-71.8297, -79.5451)
  line L24 (-71.8297, -79.5451) -> (-88.0297, -79.5451)
  line L25 (-88.0297, -79.5451) -> (-88.0297, -95.7451)
  line L26 (30.1703, -95.7451) -> (13.9703, -95.7451)
  line L27 (13.9703, -95.7451) -> (13.9703, -79.5451)
  line L28 (13.9703, -79.5451) -> (30.1703, -79.5451)
  line L29 (30.1703, -79.5451) -> (30.1703, -95.7451)
  line L30 (-86.0297, 95.2549) -> (-86.0297, -79.5451)
  line L31 (-83.5297, -79.5451) -> (-83.5297, 95.2549)
  line L32 (-71.8297, 109.4549) -> (13.9703, 109.4549)
  line L33 (13.9703, 107.4549) -> (-71.8297, 107.4549)
  line L34 (-71.8297, -93.7451) -> (13.9703, -93.7451)
  line L35 (13.9703, -91.7451) -> (-71.8297, -91.7451)
  line L36 (28.1703, 95.2549) -> (28.1703, -79.5451)
  line L37 (26.1703, -79.5451) -> (26.1703, 95.2549)
  line L38 (11.9703, 93.2549) -> (11.9703, 113.4549)
  line L39 (11.9703, 113.4549) -> (11.9703, 93.2549)
  line L40 (11.9703, 93.2549) -> (32.1703, 93.2549)
  point P0 (0, -7)
  dimension "d620" = 2
  dimension "d621" = 2
  dimension "d622" = 2
  dimension "d623" = 2
  dimension "d626" = 20.2
  dimension "d627" = 20.2
  dimension "d630" = 2
  dimension "d631" = 2.5
  dimension "d632" = 2
  dimension "d633" = 2
  dimension "d634" = 2
  dimension "d635" = 2
  dimension "d636" = 2
  dimension "d637" = 2
  dimension "d652" = 207.2
  dimension "d653" = 174.8
  dimension "d654" = 118.2
  dimension "d668" = 2
  dimension "d669" = 2
  constraints: 82 end point, 21 point on line, 17 equal length, 13 perpendicular, 8 horizontal, 5 collinear, 1 vertical
  measures "d620" distance between parallel lines of L1 L16
  measures "d621" distance between parallel lines of L0 L15
  measures "d622" distance between parallel lines of L6 L26
  measures "d623" distance between parallel lines of L3 L19
  measures "d626" distance between parallel lines of L4 L2
  measures "d627" distance between parallel lines of L3 L5
  measures "d630" distance between parallel lines of L19 L30
  measures "d631" distance between parallel lines of L30 L31
  measures "d632" distance of L20.end L32.start
  measures "d633" distance between parallel lines of L32 L33
  measures "d634" distance of L36.start L14.end
  measures "d635" distance between parallel lines of L37 L36
  measures "d636" distance between parallel lines of L35 L34
  measures "d637" distance from line of L22.end L34
  measures "d652" distance between parallel lines of L16 L26
  measures "d653" distance between parallel lines of L14 L28
  measures "d654" distance between parallel lines of L15 L19
  measures "d668" distance between parallel lines of L40 L14
  measures "d669" distance between parallel lines of L38 L17
extrude "Extrusion17" cut sketch "Sketch20" against normal blind 7.5 contours L40 L37 L14 L36 | L36 L8 L37 L40 | L14 L17 L16 L15 | L36 L28 L37 L8 | L38 L33 L5 L32 | L32 L17 L33 L38 | L28 L29 L26 L27 | L5 L33 L21 L32 | L21 L18 L19 L20 | L35 L27 L34 L7 | L7 L34 L13 L35 | L13 L34 L23 L35 | L31 L10 L30 L2 | L2 L30 L18 L31 | L23 L22 L25 L24 | L31 L24 L30 L10
sketch "Sketch21" plane through (-88.0297, 2.75, -70.5451) normal (-1, 0, 0) x (0, 0, 1)
  point P0 (70.5451, -2.75)
sketch "Sketch22" plane through (-69.8297, 2.75, 120.4549) normal (0, 0, 1) x (1, 0, 0)
  point P0 (69.8297, -2.75)
body "Solid3"
